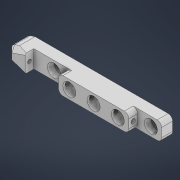
# Autodesk Inventor part: syringe tips fixture
Saved by Autodesk Inventor 2022 (Build 260153000, 153)
## iProperties
Created: 2023-04-13
Part Number: syringe tips fixture
Material: Generic
Document SubType Name: Modeling
Designer: Jakob Saugbjerg
Density: 1 g/cm^3
Appearance: Default
Author: Jakob Saugbjerg
Autodesk Inventor part; units mm, degrees
ref_plane "YZ Plane" through (0, 0, 0) normal (1, 0, 0) x (0, 1, 0)
ref_plane "XZ Plane" through (0, 0, 0) normal (0, 1, 0) x (-1, 0, 0)
ref_plane "XY Plane" through (0, 0, 0) normal (0, 0, 1) x (1, 0, 0)
sketch "Sketch1" plane through (0, 0, 0) normal (0, 0, 1) x (1, 0, 0)
  line L0 (-33, 5.5) -> (33, 5.5)
  line L1 (33, 5.5) -> (33, -5.5)
  line L2 (33, -5.5) -> (-33, -5.5)
  line L3 (-33, -5.5) -> (-33, 5.5)
  line L4 (-33, 5.5) -> (33, -5.5) construction
  line L5 (33, 5.5) -> (-33, -5.5) construction
  point P0 (0, 0)
  dimension "d0" = 66
  dimension "d1" = 11
  constraints: 12 end point, 2 midpoint, 2 parallel, 1 horizontal, 1 perpendicular
  measures "d0" distance of L1.end L2.end
  measures "d1" distance of L0.end L1.end
extrude "Extrusion1" add sketch "Sketch1" along normal blind 5
sketch "Sketch2" plane through (0, 0, 5) normal (0, 0, 1) x (1, 0, 0)
  line L0 (-33, 5.5) -> (-33, -5.5) projected
  line L1 (-33, -5.5) -> (33, -5.5) projected
  line L2 (-33, 5.5) -> (-25, 5.5)
  line L3 (-25, 5.5) -> (-25, -5.5)
  line L4 (-25, -5.5) -> (-33, -5.5)
  line L5 (-33, -5.5) -> (-33, 5.5)
  line L6 (-25, -5.5) -> (-15, -5.5)
  line L7 (33, 5.5) -> (-33, 5.5) projected
  line L8 (-15, -5.5) -> (33, -5.5)
  line L9 (33, -5.5) -> (33, 5.5)
  line L10 (33, 5.5) -> (-15, 5.5)
  line L11 (-15, 5.5) -> (-15, -5.5)
  point P0 (0, 0)
  point P1 (-15, 5.5)
  dimension "d4" = 8
  dimension "d5" = 10
  constraints: 18 end point, 4 parallel, 2 horizontal, 2 perpendicular, 2 point on line
  measures "d4" distance of L3.end L4.end
  measures "d5" distance of L3.end L6.end
extrude "Extrusion2" add sketch "Sketch2" along normal blind 4 contours L2 L3 L1 L0 | L7 L9 L1 L11
sketch "Sketch3" plane through (33, -5.5, 0) normal (1, 0, 0) x (0, 0, -1)
  line L0 (-5, 11) -> (-5, 0) projected
  line L1 (-5, 5.5) -> (-5, 7.5)
  line L2 (-5, 5.5) -> (-7, 5.5)
  circle A0 centre (-7, 5.5) radius 1
  point P0 (0, 5.5)
  dimension "d63" = 2
  dimension "d64" = 2
  dimension "d65" = 2
  constraints: 4 end point, 1 centre point, 1 coincident, 1 midpoint, 1 perpendicular, 1 point on line
  measures "d63" distance of L1.start L1.end
  measures "d64" distance of L1.start L2.end
  measures "d65" diameter of A0
extrude "Extrusion3" cut sketch "Sketch3" against normal blind 50
sketch "Sketch4" plane through (-33, -5.5, 0) normal (-1, 0, 0) x (0, 0, 1)
  line L0 (5, 0) -> (5, 11) projected
  line L1 (5, 5.5) -> (7, 5.5)
  circle A0 centre (7, 5.5) radius 0.85
  point P0 (0, 5.5)
  dimension "d66" = 2
  dimension "d104" = 1.7
  constraints: 2 end point, 1 centre point, 1 coincident, 1 horizontal, 1 midpoint
  measures "d66" distance of L1.start L1.end
  measures "d104" diameter of A0
extrude "Extrusion4" cut sketch "Sketch4" against normal blind 15
sketch "Sketch13" plane through (0, 0, 9) normal (0, 0, 1) x (1, 0, 0)
  line L0 (-33, 5.5) -> (-33, -5.5) projected
  line L1 (-33, 0.8) -> (-25, 0.8) projected
  line L2 (-33, 0) -> (-33, 2.8)
  line L3 (-15, 5.5) -> (-25, 5.5) projected
  line L4 (-33, 2.8) -> (-25, 5.5)
  line L5 (-33, 0) -> (-33, -2.8)
  line L6 (-25, -5.5) -> (-15, -5.5) projected
  line L7 (-33, -2.8) -> (-25, -5.5)
  line L8 (-25, -5.5) -> (-25, 5.5)
  line L9 (-25, 5.5) -> (-33, 5.5)
  line L10 (-33, -5.5) -> (-25, -5.5) projected
  line L11 (-33, -2.8) -> (-33, -5.5)
  line L12 (-33, -5.5) -> (-25, -5.5)
  point P0 (0, 0)
  dimension "d68" = 2.8
  dimension "d69" = 2.8
  constraints: 16 end point, 2 point on line, 1 collinear, 1 horizontal, 1 midpoint, 1 parallel, 1 vertical
  measures "d68" distance of L2.start L2.end
  measures "d69" distance of L2.start L5.end
extrude "Extrusion12" cut sketch "Sketch13" against normal blind 15 contours L9 L4 L0 | L10 L0 L7
fillet "Fillet5" radius 2 2 edges at (-33, 2.8, 4.5) (-33, -2.8, 4.5)
chamfer "Chamfer1" distance 2 angle 45 5 edges at (-32.6247, -2.5305, 9) (-33, 0, 9) (-32.6247, 2.5305, 9) (-28.3198, 4.3796, 9) (-28.3198, -4.3796, 9)
sketch "Sketch14" plane through (0, 0, 9) normal (0, 0, 1) x (1, 0, 0)
  line L0 (33, 1) -> (33, -1) projected
  line L1 (33, 0) -> (28.15, 0)
  circle A0 centre (28.15, 0) radius 1.75
  circle A1 centre (17.15, 0) radius 1.75
  circle A2 centre (6.15, 0) radius 1.75
  circle A3 centre (-4.85, 0) radius 1.75
  circle A4 centre (-15.85, 0) radius 1.75
  point P0 (0, 0)
  dimension "d76" = 4.85
  dimension "d77" = 3.5
  dimension "d80" = 11
  constraints: 5 centre point, 2 end point, 2 horizontal, 1 coincident, 1 midpoint, 8 other
  measures "d76" distance of L1.start L1.end
  measures "d77" diameter of A0
  measures "d80" distance of A0.centre A1.centre
extrude "Extrusion13" cut sketch "Sketch14" against normal blind 15
sketch "Sketch15" plane through (0, 0, 9) normal (0, 0, 1) x (1, 0, 0)
  line L0 (33, -5.5) -> (33, 5.5) projected
  line L1 (33, 5.5) -> (-34.6652, 5.5)
  line L2 (-34.6652, 5.5) -> (-34.6652, 4)
  line L3 (-34.6652, 4) -> (33, 4)
  line L4 (33, 4) -> (33, 5.5)
  line L5 (-25, -5.5) -> (33, -5.5) projected
  line L6 (33, -5.5) -> (-34.6652, -5.5)
  line L7 (-34.6652, -5.5) -> (-34.6652, -4)
  line L8 (-34.6652, -4) -> (33, -4)
  line L9 (33, -4) -> (33, -5.5)
  point P0 (0, 0)
  point P1 (33, 4)
  dimension "d87" = 1.5
  dimension "d88" = 1.5
  constraints: 16 end point, 4 parallel, 2 horizontal, 2 perpendicular, 1 point on line
  measures "d87" distance of L2.end L1.end
  measures "d88" distance of L6.end L7.end
extrude "Extrusion14" cut sketch "Sketch15" against normal blind 15
sketch "Sketch16" plane through (0, 0, 9) normal (0, 0, 1) x (1, 0, 0)
  circle A0 centre (-4.85, 0) radius 1.75 projected
  circle A1 centre (-4.85, 0) radius 2.95
  line L0 (-7.8, 0) -> (-9.8, 0)
  line L1 (-9.8, 0) -> (-9.8, 4)
  line L2 (-29.4444, 4) -> (33, 4) projected
  line L3 (-15, -1.5297) -> (-15, -4) projected
  line L4 (-9.8, 4) -> (-15, 4)
  line L5 (-15, 4) -> (-15, -4)
  line L6 (-15, -4) -> (-9.8, -4)
  line L7 (-9.8, -4) -> (-9.8, 4)
  circle A2 centre (17.15, 0) radius 1.75 projected
  circle A3 centre (17.15, 0) radius 2.95
  line L8 (20.1, 0) -> (22.1, 0)
  line L9 (22.1, 0) -> (22.1, 4)
  line L10 (33, -4) -> (33, 4) projected
  line L11 (22.1, 4) -> (33, 4)
  line L12 (33, 4) -> (33, -4)
  line L13 (33, -4) -> (22.1, -4)
  line L14 (22.1, -4) -> (22.1, 4)
  point P0 (0, 0)
  dimension "d91" = 5.9
  dimension "d93" = 5.9
  dimension "d92" = 2
  dimension "d94" = 2
  constraints: 24 end point, 4 horizontal, 4 parallel, 3 perpendicular, 2 coincident, 2 horizontal alignment, 2 point on line, 1 vertical, 4 other
  measures "d92" distance of L0.start L0.end
  measures "d94" distance of L8.start L8.end
extrude "Extrusion15" cut sketch "Sketch16" against normal blind 4 contours L7 L6 L3 L5 L2 L1 | L2 L10 L13 L14 L9
sketch "Sketch17" plane through (0, 0, 5) normal (0, 0, 1) x (1, 0, 0)
  circle A0 centre (28.15, 0) radius 1.75 projected
  circle A1 centre (28.15, 0) radius 2.95
  circle A2 centre (-15.85, 0) radius 1.75 projected
  circle A3 centre (-15.85, 0) radius 2.95
  circle A4 centre (17.15, 0) radius 1.75 projected
  circle A5 centre (17.15, 0) radius 2.95
  circle A6 centre (6.15, 0) radius 1.75 projected
  circle A7 centre (6.15, 0) radius 2.95
  circle A8 centre (-4.85, 0) radius 1.75 projected
  circle A9 centre (-4.85, 0) radius 2.95
  point P0 (0, 0)
  dimension "d97" = 5.9
  dimension "d98" = 5.9
  constraints: 5 centre point, 5 coincident
  measures "d97" diameter of A1
  measures "d98" diameter of A3
extrude "Extrusion16" cut sketch "Sketch17" along normal blind 8 and the other way blind 3 contours A0 | A1 | A2 | A3 | A4 | A5 | A6 | A7 | A8 | A9
fillet "Fillet6" radius 2 6 edges at (33, -4, 2.5) (33, 4, 2.5) (22.1, -4, 7) (22.1, 4, 7) (-9.8, -4, 7) (-9.8, 4, 7)
body "Solid1"
